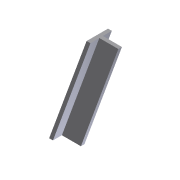
# Autodesk Inventor part: brace
Saved by Autodesk Inventor 2012 (Build 160160000, 160)
## iProperties
Created: 2012-04-25
Part Number: brace
Material: Default
Document SubType Name: Modeling
Designer: Antonella Wilby
Density: 1 g/cm^3
Author: Antonella Wilby
Autodesk Inventor part; units mm, degrees
ref_plane "YZ Plane" through (0, 0, 0) normal (1, 0, 0) x (0, 1, 0)
ref_plane "XZ Plane" through (0, 0, 0) normal (0, 1, 0) x (-1, 0, 0)
ref_plane "XY Plane" through (0, 0, 0) normal (0, 0, 1) x (1, 0, 0)
sketch "Sketch1" plane through (0, 0, 0) normal (0, 0, 1) x (1, 0, 0)
  line L0 (-30.9834, 0) -> (43.9922, 0) projected
  line L1 (0, -18.288) -> (0, 109.728) projected
  line L2 (0, 0) -> (33.2814, 91.44)
  line L3 (33.2814, 91.44) -> (13.0089, 91.44)
  line L4 (13.0089, 91.44) -> (-20.2726, 0)
  dimension "d0" = 19.05
  dimension "d10" = 20
  dimension "d11" = 91.44
  constraints: 6 end point, 1 parallel, 1 perpendicular, 1 point on line
  measures "d0" distance between parallel lines of L2 L4
  measures "d10" angle of L1 L2
  measures "d11" distance between parallel lines of L3 L0
extrude "Extrusion1" add sketch "Sketch1" along normal mid plane 19.05
sketch "Sketch3" plane through (0, 0, 9.525) normal (0, 0, 1) x (1, 0, 0)
  line L0 (-20.2726, 0) -> (13.0089, 91.44) projected
  line L1 (0, 0) -> (-20.2726, 0) projected
  line L2 (33.2814, 91.44) -> (0, 0) projected
  line L3 (13.0089, 91.44) -> (33.2814, 91.44) projected
  line L4 (-16.8938, 0) -> (16.3876, 91.44)
  dimension "d7" = 3.175
  constraints: 2 end point, 2 point on line
  measures "d7" distance between parallel lines of L0 L4
extrude "Extrusion2" cut sketch "Sketch3" against normal blind 7.9375 contours L4 L3 L2 L1
mirror "Mirror1" about plane through (0, 0, 0) normal (0, 0, 1) of "Extrusion2"
body "Solid1"
